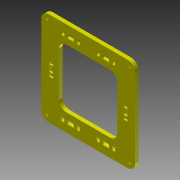
# Autodesk Inventor part: base
Saved by Autodesk Inventor 2012 SP1 (Build 160190100, 190)
## iProperties
Created: 2011-10-14
Part Number: base
Document SubType Name: Modeling
Designer: cramera
Density: 0.952 g/cm^3
Material: High Density Polyethylene
Mass: 589.682 g
Surface Area: 1422.26 cm^2
Volume: 619.414 cm^3
Autodesk Inventor part; units mm, degrees
ref_plane "YZ Plane" through (0, 0, 0) normal (1, 0, 0) x (0, 1, 0)
ref_plane "XZ Plane" through (0, 0, 0) normal (0, 1, 0) x (-1, 0, 0)
ref_plane "XY Plane" through (0, 0, 0) normal (0, 0, 1) x (1, 0, 0)
derived "skeleton.ipt"
sketch "POCKET_1-4" plane through (0, 0, 0) normal (0, 0, 1) x (1, 0, 0)
  line L0 (756.4523, 867.4563) -> (756.4523, 854.7563)
  arc A0 (791.01, 767.5708) -> (789.4225, 769.1583) centre (789.4225, 767.5708) ccw
  arc A1 (683.1733, 854.7563) -> (684.7608, 853.1688) centre (684.7608, 854.7563) ccw
  line L1 (683.1733, 854.7563) -> (683.1733, 867.4563)
  arc A2 (684.7608, 869.0438) -> (683.1733, 867.4563) centre (684.7608, 867.4563) ccw
  line L2 (684.7608, 869.0438) -> (754.8648, 869.0438)
  line L3 (756.4523, 613.4563) -> (756.4523, 626.1563)
  arc A3 (684.7608, 627.7438) -> (683.1733, 626.1563) centre (684.7608, 626.1563) ccw
  line L4 (683.1733, 626.1563) -> (683.1733, 613.4563)
  arc A4 (683.1733, 613.4563) -> (684.7608, 611.8688) centre (684.7608, 613.4563) ccw
  line L5 (684.7608, 611.8688) -> (754.8648, 611.8688)
  arc A5 (754.8648, 611.8688) -> (756.4523, 613.4563) centre (754.8648, 613.4563) ccw
  arc A6 (756.4523, 867.4563) -> (754.8648, 869.0438) centre (754.8648, 867.4563) ccw
  arc A7 (756.4523, 626.1563) -> (754.8648, 627.7438) centre (754.8648, 626.1563) ccw
  line L6 (754.8648, 627.7438) -> (684.7608, 627.7438)
  arc A8 (789.4225, 711.7543) -> (791.01, 713.3418) centre (789.4225, 713.3418) ccw
  line L7 (789.4225, 711.7543) -> (776.7225, 711.7543)
  arc A9 (775.135, 713.3418) -> (776.7225, 711.7543) centre (776.7225, 713.3418) ccw
  line L8 (775.135, 713.3418) -> (775.135, 767.5708)
  arc A10 (776.7225, 769.1583) -> (775.135, 767.5708) centre (776.7225, 767.5708) ccw
  line L9 (776.7225, 769.1583) -> (789.4225, 769.1583)
  line L10 (791.01, 767.5708) -> (791.01, 713.3418)
  arc A11 (568.3926, 613.4563) -> (569.9801, 611.8688) centre (569.9801, 613.4563) ccw
  line L11 (568.3926, 613.4563) -> (568.3926, 626.1563)
  arc A12 (569.9801, 627.7438) -> (568.3926, 626.1563) centre (569.9801, 626.1563) ccw
  line L12 (569.9801, 627.7438) -> (640.0841, 627.7438)
  arc A13 (641.6716, 626.1563) -> (640.0841, 627.7438) centre (640.0841, 626.1563) ccw
  line L13 (641.6716, 626.1563) -> (641.6716, 613.4563)
  arc A14 (640.0841, 611.8688) -> (641.6716, 613.4563) centre (640.0841, 613.4563) ccw
  line L14 (640.0841, 611.8688) -> (569.9801, 611.8688)
  arc A15 (641.6716, 867.4563) -> (640.0841, 869.0438) centre (640.0841, 867.4563) ccw
  line L15 (640.0841, 869.0438) -> (569.9801, 869.0438)
  arc A16 (569.9801, 869.0438) -> (568.3926, 867.4563) centre (569.9801, 867.4563) ccw
  line L16 (568.3926, 867.4563) -> (568.3926, 854.7563)
  arc A17 (568.3926, 854.7563) -> (569.9801, 853.1688) centre (569.9801, 854.7563) ccw
  line L17 (569.9801, 853.1688) -> (640.0841, 853.1688)
  arc A18 (640.0841, 853.1688) -> (641.6716, 854.7563) centre (640.0841, 854.7563) ccw
  line L18 (641.6716, 854.7563) -> (641.6716, 867.4563)
  arc A19 (533.835, 713.3418) -> (535.4225, 711.7543) centre (535.4225, 713.3418) ccw
  line L19 (535.4225, 711.7543) -> (548.1225, 711.7543)
  arc A20 (548.1225, 711.7543) -> (549.71, 713.3418) centre (548.1225, 713.3418) ccw
  line L20 (549.71, 713.3418) -> (549.71, 767.5708)
  arc A21 (549.71, 767.5708) -> (548.1225, 769.1583) centre (548.1225, 767.5708) ccw
  line L21 (548.1225, 769.1583) -> (535.4225, 769.1583)
  arc A22 (535.4225, 769.1583) -> (533.835, 767.5708) centre (535.4225, 767.5708) ccw
  line L22 (533.835, 767.5708) -> (533.835, 713.3418)
  arc A23 (754.8648, 853.1688) -> (756.4523, 854.7563) centre (754.8648, 854.7563) ccw
  line L23 (754.8648, 853.1688) -> (684.7608, 853.1688)
  constraints: 48 end point, 48 point on circle, 24 centre point
sketch "STOCK_12MM" plane through (0, 0, 0) normal (0, 0, 1) x (1, 0, 0)
  line L0 (457.2, 0) -> (914.4, 0)
  line L1 (914.4, 0) -> (914.4, 914.4)
  line L2 (914.4, 914.4) -> (457.2, 914.4)
  line L3 (457.2, 914.4) -> (457.2, 0)
  line L4 (457.2, 0) -> (457.2, 914.4)
  constraints: 10 end point
sketch "THROUGH-CUT" plane through (0, 0, 0) normal (0, 0, 1) x (1, 0, 0)
  arc A0 (777.1035, 720.3494) -> (779.3485, 718.1043) centre (778.226, 719.2268) ccw
  line L0 (779.3485, 718.1043) -> (787.1774, 718.1043)
  arc A1 (787.1774, 718.1043) -> (789.4225, 720.3494) centre (788.2999, 719.2268) ccw
  line L1 (789.4225, 720.3494) -> (789.4225, 726.0192)
  arc A2 (594.5546, 613.4563) -> (596.7997, 613.4563) centre (595.6772, 614.5788) ccw
  line L2 (596.7997, 613.4563) -> (613.2646, 613.4563)
  arc A3 (613.2646, 613.4563) -> (615.5096, 613.4563) centre (614.3871, 614.5788) ccw
  arc A4 (615.5096, 613.4563) -> (615.5096, 615.7014) centre (614.3871, 614.5788) ccw
  line L3 (615.5096, 615.7014) -> (615.5096, 623.5302)
  arc A5 (615.5096, 623.5302) -> (615.5096, 625.7753) centre (614.3871, 624.6528) ccw
  arc A6 (615.5096, 625.7753) -> (613.2646, 625.7753) centre (614.3871, 624.6528) ccw
  line L4 (613.2646, 625.7753) -> (596.7997, 625.7753)
  arc A7 (596.7997, 625.7753) -> (594.5546, 623.5302) centre (595.6772, 624.6528) ccw
  line L5 (594.5546, 623.5302) -> (594.5546, 615.7014)
  arc A8 (594.5546, 615.7014) -> (594.5546, 613.4563) centre (595.6772, 614.5788) ccw
  arc A9 (728.0452, 613.4563) -> (730.2903, 613.4563) centre (729.1678, 614.5788) ccw
  line L6 (728.0452, 613.4563) -> (711.5804, 613.4563)
  arc A10 (709.3353, 613.4563) -> (711.5804, 613.4563) centre (710.4578, 614.5788) ccw
  arc A11 (709.3353, 615.7014) -> (709.3353, 613.4563) centre (710.4578, 614.5788) ccw
  line L7 (709.3353, 615.7014) -> (709.3353, 623.5302)
  arc A12 (709.3353, 625.7753) -> (709.3353, 623.5302) centre (710.4578, 624.6528) ccw
  arc A13 (711.5804, 625.7753) -> (709.3353, 625.7753) centre (710.4578, 624.6528) ccw
  line L8 (711.5804, 625.7753) -> (728.0452, 625.7753)
  arc A14 (730.2903, 623.5302) -> (728.0452, 625.7753) centre (729.1678, 624.6528) ccw
  line L9 (730.2903, 623.5302) -> (730.2903, 615.7014)
  arc A15 (730.2903, 613.4563) -> (730.2903, 615.7014) centre (729.1678, 614.5788) ccw
  arc A16 (625.1616, 855.1373) -> (627.4067, 855.1373) centre (626.2842, 856.2598) ccw
  arc A17 (625.1616, 857.3824) -> (625.1616, 855.1373) centre (626.2842, 856.2598) ccw
  line L10 (625.1616, 857.3824) -> (625.1616, 865.2112)
  arc A18 (625.1616, 867.4563) -> (625.1616, 865.2112) centre (626.2842, 866.3338) ccw
  arc A19 (627.4067, 867.4563) -> (625.1616, 867.4563) centre (626.2842, 866.3338) ccw
  line L11 (627.4067, 867.4563) -> (633.0766, 867.4563)
  arc A20 (635.3216, 867.4563) -> (633.0766, 867.4563) centre (634.1991, 866.3338) ccw
  arc A21 (635.3216, 865.2112) -> (635.3216, 867.4563) centre (634.1991, 866.3338) ccw
  line L12 (635.3216, 865.2112) -> (635.3216, 857.3824)
  arc A22 (635.3216, 855.1373) -> (635.3216, 857.3824) centre (634.1991, 856.2598) ccw
  arc A23 (633.0766, 855.1373) -> (635.3216, 855.1373) centre (634.1991, 856.2598) ccw
  line L13 (633.0766, 855.1373) -> (627.4067, 855.1373)
  arc A24 (627.4067, 625.7753) -> (625.1616, 625.7753) centre (626.2842, 624.6528) ccw
  arc A25 (625.1616, 625.7753) -> (625.1616, 623.5302) centre (626.2842, 624.6528) ccw
  line L14 (625.1616, 623.5302) -> (625.1616, 615.7014)
  arc A26 (625.1616, 615.7014) -> (625.1616, 613.4563) centre (626.2842, 614.5788) ccw
  arc A27 (625.1616, 613.4563) -> (627.4067, 613.4563) centre (626.2842, 614.5788) ccw
  line L15 (627.4067, 613.4563) -> (633.0766, 613.4563)
  arc A28 (633.0766, 613.4563) -> (635.3216, 613.4563) centre (634.1991, 614.5788) ccw
  arc A29 (635.3216, 613.4563) -> (635.3216, 615.7014) centre (634.1991, 614.5788) ccw
  line L16 (635.3216, 615.7014) -> (635.3216, 623.5302)
  arc A30 (635.3216, 623.5302) -> (635.3216, 625.7753) centre (634.1991, 624.6528) ccw
  arc A31 (635.3216, 625.7753) -> (633.0766, 625.7753) centre (634.1991, 624.6528) ccw
  line L17 (633.0766, 625.7753) -> (627.4067, 625.7753)
  arc A32 (697.4382, 855.1373) -> (699.6833, 855.1373) centre (698.5608, 856.2598) ccw
  arc A33 (699.6833, 855.1373) -> (699.6833, 857.3824) centre (698.5608, 856.2598) ccw
  line L18 (699.6833, 857.3824) -> (699.6833, 865.2112)
  arc A34 (699.6833, 865.2112) -> (699.6833, 867.4563) centre (698.5608, 866.3338) ccw
  arc A35 (699.6833, 867.4563) -> (697.4382, 867.4563) centre (698.5608, 866.3338) ccw
  line L19 (697.4382, 867.4563) -> (691.7684, 867.4563)
  arc A36 (691.7684, 867.4563) -> (689.5233, 867.4563) centre (690.6458, 866.3338) ccw
  arc A37 (689.5233, 867.4563) -> (689.5233, 865.2112) centre (690.6458, 866.3338) ccw
  line L20 (689.5233, 865.2112) -> (689.5233, 857.3824)
  arc A38 (689.5233, 857.3824) -> (689.5233, 855.1373) centre (690.6458, 856.2598) ccw
  arc A39 (689.5233, 855.1373) -> (691.7684, 855.1373) centre (690.6458, 856.2598) ccw
  line L21 (691.7684, 855.1373) -> (697.4382, 855.1373)
  arc A40 (574.7426, 857.3824) -> (574.7426, 855.1373) centre (575.8652, 856.2598) ccw
  line L22 (574.7426, 857.3824) -> (574.7426, 865.2112)
  arc A41 (574.7426, 867.4563) -> (574.7426, 865.2112) centre (575.8652, 866.3338) ccw
  arc A42 (576.9877, 867.4563) -> (574.7426, 867.4563) centre (575.8652, 866.3338) ccw
  line L23 (576.9877, 867.4563) -> (582.6576, 867.4563)
  arc A43 (584.9026, 867.4563) -> (582.6576, 867.4563) centre (583.7801, 866.3338) ccw
  arc A44 (584.9026, 865.2112) -> (584.9026, 867.4563) centre (583.7801, 866.3338) ccw
  line L24 (584.9026, 865.2112) -> (584.9026, 857.3824)
  arc A45 (584.9026, 855.1373) -> (584.9026, 857.3824) centre (583.7801, 856.2598) ccw
  arc A46 (582.6576, 855.1373) -> (584.9026, 855.1373) centre (583.7801, 856.2598) ccw
  line L25 (582.6576, 855.1373) -> (576.9877, 855.1373)
  arc A47 (574.7426, 855.1373) -> (576.9877, 855.1373) centre (575.8652, 856.2598) ccw
  arc A48 (750.1023, 855.1373) -> (750.1023, 857.3824) centre (748.9798, 856.2598) ccw
  line L26 (750.1023, 857.3824) -> (750.1023, 865.2112)
  arc A49 (750.1023, 865.2112) -> (750.1023, 867.4563) centre (748.9798, 866.3338) ccw
  arc A50 (750.1023, 867.4563) -> (747.8572, 867.4563) centre (748.9798, 866.3338) ccw
  line L27 (747.8572, 867.4563) -> (742.1874, 867.4563)
  arc A51 (742.1874, 867.4563) -> (739.9423, 867.4563) centre (741.0648, 866.3338) ccw
  arc A52 (739.9423, 867.4563) -> (739.9423, 865.2112) centre (741.0648, 866.3338) ccw
  arc A53 (545.4964, 718.1043) -> (547.7415, 720.3494) centre (546.6189, 719.2268) ccw
  arc A54 (739.9423, 857.3824) -> (739.9423, 855.1373) centre (741.0648, 856.2598) ccw
  arc A55 (739.9423, 855.1373) -> (742.1874, 855.1373) centre (741.0648, 856.2598) ccw
  line L28 (742.1874, 855.1373) -> (747.8572, 855.1373)
  arc A56 (747.8572, 855.1373) -> (750.1023, 855.1373) centre (748.9798, 856.2598) ccw
  arc A57 (750.1023, 623.5302) -> (750.1023, 625.7753) centre (748.9798, 624.6528) ccw
  line L29 (750.1023, 623.5302) -> (750.1023, 615.7014)
  arc A58 (750.1023, 613.4563) -> (750.1023, 615.7014) centre (748.9798, 614.5788) ccw
  arc A59 (747.8572, 613.4563) -> (750.1023, 613.4563) centre (748.9798, 614.5788) ccw
  line L30 (747.8572, 613.4563) -> (742.1874, 613.4563)
  arc A60 (739.9423, 613.4563) -> (742.1874, 613.4563) centre (741.0648, 614.5788) ccw
  arc A61 (739.9423, 615.7014) -> (739.9423, 613.4563) centre (741.0648, 614.5788) ccw
  line L31 (739.9423, 615.7014) -> (739.9423, 623.5302)
  arc A62 (739.9423, 625.7753) -> (739.9423, 623.5302) centre (741.0648, 624.6528) ccw
  arc A63 (742.1874, 625.7753) -> (739.9423, 625.7753) centre (741.0648, 624.6528) ccw
  line L32 (742.1874, 625.7753) -> (747.8572, 625.7753)
  arc A64 (750.1023, 625.7753) -> (747.8572, 625.7753) centre (748.9798, 624.6528) ccw
  circle A65 centre (527.8454, 605.8792) radius 3.175
  arc A66 (574.7426, 625.7753) -> (574.7426, 623.5302) centre (575.8652, 624.6528) ccw
  line L33 (574.7426, 623.5302) -> (574.7426, 615.7014)
  arc A67 (574.7426, 615.7014) -> (574.7426, 613.4563) centre (575.8652, 614.5788) ccw
  arc A68 (574.7426, 613.4563) -> (576.9877, 613.4563) centre (575.8652, 614.5788) ccw
  line L34 (576.9877, 613.4563) -> (582.6576, 613.4563)
  arc A69 (582.6576, 613.4563) -> (584.9026, 613.4563) centre (583.7801, 614.5788) ccw
  arc A70 (584.9026, 613.4563) -> (584.9026, 615.7014) centre (583.7801, 614.5788) ccw
  line L35 (584.9026, 615.7014) -> (584.9026, 623.5302)
  arc A71 (584.9026, 623.5302) -> (584.9026, 625.7753) centre (583.7801, 624.6528) ccw
  arc A72 (584.9026, 625.7753) -> (582.6576, 625.7753) centre (583.7801, 624.6528) ccw
  line L36 (582.6576, 625.7753) -> (576.9877, 625.7753)
  arc A73 (576.9877, 625.7753) -> (574.7426, 625.7753) centre (575.8652, 624.6528) ccw
  circle A74 centre (796.9996, 875.0334) radius 3.175
  arc A75 (596.7997, 867.4563) -> (594.5546, 867.4563) centre (595.6772, 866.3338) ccw
  line L37 (596.7997, 867.4563) -> (613.2646, 867.4563)
  arc A76 (615.5096, 867.4563) -> (613.2646, 867.4563) centre (614.3871, 866.3338) ccw
  arc A77 (615.5096, 865.2112) -> (615.5096, 867.4563) centre (614.3871, 866.3338) ccw
  line L38 (615.5096, 865.2112) -> (615.5096, 857.3824)
  arc A78 (615.5096, 855.1373) -> (615.5096, 857.3824) centre (614.3871, 856.2598) ccw
  arc A79 (613.2646, 855.1373) -> (615.5096, 855.1373) centre (614.3871, 856.2598) ccw
  line L39 (613.2646, 855.1373) -> (596.7997, 855.1373)
  arc A80 (594.5546, 857.3824) -> (596.7997, 855.1373) centre (595.6772, 856.2598) ccw
  line L40 (594.5546, 857.3824) -> (594.5546, 865.2112)
  arc A81 (594.5546, 867.4563) -> (594.5546, 865.2112) centre (595.6772, 866.3338) ccw
  circle A82 centre (527.8454, 875.0334) radius 3.175
  circle A83 centre (796.9996, 605.8792) radius 3.175
  line L41 (787.1774, 762.8083) -> (779.3485, 762.8083)
  arc A84 (779.3485, 762.8083) -> (777.1035, 760.5632) centre (778.226, 761.6858) ccw
  line L42 (777.1035, 760.5632) -> (777.1035, 754.8934)
  arc A85 (777.1035, 754.8934) -> (777.1035, 752.6483) centre (778.226, 753.7708) ccw
  arc A86 (777.1035, 752.6483) -> (779.3485, 752.6483) centre (778.226, 753.7708) ccw
  line L43 (779.3485, 752.6483) -> (787.1774, 752.6483)
  arc A87 (787.1774, 752.6483) -> (789.4225, 752.6483) centre (788.2999, 753.7708) ccw
  arc A88 (789.4225, 752.6483) -> (789.4225, 754.8934) centre (788.2999, 753.7708) ccw
  line L44 (789.4225, 754.8934) -> (789.4225, 760.5632)
  arc A89 (789.4225, 760.5632) -> (787.1774, 762.8083) centre (788.2999, 761.6858) ccw
  line L45 (732.2725, 835.7063) -> (592.5725, 835.7063)
  arc A90 (592.5725, 835.7063) -> (567.1725, 810.3063) centre (592.5725, 810.3063) ccw
  line L46 (567.1725, 810.3063) -> (567.1725, 670.6063)
  arc A91 (567.1725, 670.6063) -> (592.5725, 645.2063) centre (592.5725, 670.6063) ccw
  line L47 (592.5725, 645.2063) -> (732.2725, 645.2063)
  arc A92 (732.2725, 645.2063) -> (757.6725, 670.6063) centre (732.2725, 670.6063) ccw
  line L48 (757.6725, 670.6063) -> (757.6725, 810.3063)
  arc A93 (757.6725, 810.3063) -> (732.2725, 835.7063) centre (732.2725, 810.3063) ccw
  line L49 (547.7415, 747.1012) -> (547.7415, 733.8114)
  arc A94 (547.7415, 731.5663) -> (547.7415, 733.8114) centre (546.6189, 732.6888) ccw
  arc A95 (545.4964, 731.5663) -> (547.7415, 731.5663) centre (546.6189, 732.6888) ccw
  line L50 (545.4964, 731.5663) -> (537.6675, 731.5663)
  arc A96 (535.4225, 731.5663) -> (537.6675, 731.5663) centre (536.545, 732.6888) ccw
  arc A97 (535.4225, 733.8114) -> (535.4225, 731.5663) centre (536.545, 732.6888) ccw
  arc A98 (730.2903, 867.4563) -> (728.0452, 867.4563) centre (729.1678, 866.3338) ccw
  arc A99 (537.6675, 749.3463) -> (535.4225, 747.1012) centre (536.545, 748.2238) ccw
  line L51 (537.6675, 749.3463) -> (545.4964, 749.3463)
  arc A100 (547.7415, 747.1012) -> (545.4964, 749.3463) centre (546.6189, 748.2238) ccw
  line L52 (728.0452, 867.4563) -> (711.5804, 867.4563)
  arc A101 (711.5804, 867.4563) -> (709.3353, 867.4563) centre (710.4578, 866.3338) ccw
  arc A102 (709.3353, 867.4563) -> (709.3353, 865.2112) centre (710.4578, 866.3338) ccw
  line L53 (709.3353, 865.2112) -> (709.3353, 857.3824)
  line L54 (777.1035, 747.1012) -> (777.1035, 733.8114)
  arc A103 (777.1035, 733.8114) -> (777.1035, 731.5663) centre (778.226, 732.6888) ccw
  arc A104 (777.1035, 731.5663) -> (779.3485, 731.5663) centre (778.226, 732.6888) ccw
  line L55 (779.3485, 731.5663) -> (787.1774, 731.5663)
  arc A105 (787.1774, 731.5663) -> (789.4225, 731.5663) centre (788.2999, 732.6888) ccw
  arc A106 (789.4225, 731.5663) -> (789.4225, 733.8114) centre (788.2999, 732.6888) ccw
  line L56 (789.4225, 733.8114) -> (789.4225, 747.1012)
  arc A107 (789.4225, 747.1012) -> (787.1774, 749.3463) centre (788.2999, 748.2238) ccw
  line L57 (787.1774, 749.3463) -> (779.3485, 749.3463)
  arc A108 (779.3485, 749.3463) -> (777.1035, 747.1012) centre (778.226, 748.2238) ccw
  arc A109 (709.3353, 857.3824) -> (709.3353, 855.1373) centre (710.4578, 856.2598) ccw
  arc A110 (709.3353, 855.1373) -> (711.5804, 855.1373) centre (710.4578, 856.2598) ccw
  line L58 (711.5804, 855.1373) -> (728.0452, 855.1373)
  arc A111 (728.0452, 855.1373) -> (730.2903, 857.3824) centre (729.1678, 856.2598) ccw
  line L59 (730.2903, 857.3824) -> (730.2903, 865.2112)
  arc A112 (730.2903, 865.2112) -> (730.2903, 867.4563) centre (729.1678, 866.3338) ccw
  line L60 (537.6675, 762.8083) -> (545.4964, 762.8083)
  arc A113 (547.7415, 760.5632) -> (545.4964, 762.8083) centre (546.6189, 761.6858) ccw
  line L61 (547.7415, 760.5632) -> (547.7415, 754.8934)
  arc A114 (547.7415, 752.6483) -> (547.7415, 754.8934) centre (546.6189, 753.7708) ccw
  arc A115 (545.4964, 752.6483) -> (547.7415, 752.6483) centre (546.6189, 753.7708) ccw
  line L62 (545.4964, 752.6483) -> (537.6675, 752.6483)
  arc A116 (535.4225, 752.6483) -> (537.6675, 752.6483) centre (536.545, 753.7708) ccw
  arc A117 (535.4225, 754.8934) -> (535.4225, 752.6483) centre (536.545, 753.7708) ccw
  line L63 (535.4225, 754.8934) -> (535.4225, 760.5632)
  line L64 (739.9423, 865.2112) -> (739.9423, 857.3824)
  arc A118 (537.6675, 762.8083) -> (535.4225, 760.5632) centre (536.545, 761.6858) ccw
  line L65 (535.4225, 588.0563) -> (789.4225, 588.0563)
  arc A119 (789.4225, 588.0563) -> (814.8225, 613.4563) centre (789.4225, 613.4563) ccw
  line L66 (814.8225, 613.4563) -> (814.8225, 867.4563)
  arc A120 (814.8225, 867.4563) -> (789.4225, 892.8563) centre (789.4225, 867.4563) ccw
  line L67 (789.4225, 892.8563) -> (535.4225, 892.8563)
  arc A121 (535.4225, 892.8563) -> (510.0225, 867.4563) centre (535.4225, 867.4563) ccw
  line L68 (510.0225, 867.4563) -> (510.0225, 613.4563)
  arc A122 (510.0225, 613.4563) -> (535.4225, 588.0563) centre (535.4225, 613.4563) ccw
  arc A123 (537.6675, 728.2643) -> (535.4225, 726.0192) centre (536.545, 727.1418) ccw
  line L69 (537.6675, 728.2643) -> (545.4964, 728.2643)
  arc A124 (547.7415, 726.0192) -> (545.4964, 728.2643) centre (546.6189, 727.1418) ccw
  line L70 (547.7415, 726.0192) -> (547.7415, 720.3494)
  line L71 (545.4964, 718.1043) -> (537.6675, 718.1043)
  arc A125 (535.4225, 720.3494) -> (537.6675, 718.1043) centre (536.545, 719.2268) ccw
  line L72 (535.4225, 720.3494) -> (535.4225, 726.0192)
  arc A126 (699.6833, 625.7753) -> (697.4382, 625.7753) centre (698.5608, 624.6528) ccw
  arc A127 (699.6833, 623.5302) -> (699.6833, 625.7753) centre (698.5608, 624.6528) ccw
  line L73 (699.6833, 623.5302) -> (699.6833, 615.7014)
  arc A128 (699.6833, 613.4563) -> (699.6833, 615.7014) centre (698.5608, 614.5788) ccw
  arc A129 (697.4382, 613.4563) -> (699.6833, 613.4563) centre (698.5608, 614.5788) ccw
  line L74 (697.4382, 613.4563) -> (691.7684, 613.4563)
  arc A130 (689.5233, 613.4563) -> (691.7684, 613.4563) centre (690.6458, 614.5788) ccw
  arc A131 (689.5233, 615.7014) -> (689.5233, 613.4563) centre (690.6458, 614.5788) ccw
  line L75 (689.5233, 615.7014) -> (689.5233, 623.5302)
  arc A132 (689.5233, 625.7753) -> (689.5233, 623.5302) centre (690.6458, 624.6528) ccw
  arc A133 (691.7684, 625.7753) -> (689.5233, 625.7753) centre (690.6458, 624.6528) ccw
  line L76 (691.7684, 625.7753) -> (697.4382, 625.7753)
  arc A134 (789.4225, 726.0192) -> (787.1774, 728.2643) centre (788.2999, 727.1418) ccw
  line L77 (787.1774, 728.2643) -> (779.3485, 728.2643)
  arc A135 (779.3485, 728.2643) -> (777.1035, 726.0192) centre (778.226, 727.1418) ccw
  line L78 (777.1035, 726.0192) -> (777.1035, 720.3494)
  line L79 (535.4225, 733.8114) -> (535.4225, 747.1012)
  constraints: 264 point on circle, 160 end point, 136 centre point
extrude "Extrusion1" add sketch "THROUGH-CUT" along normal blind 12
extrude "Extrusion2" cut sketch "POCKET_1-4" along normal blind 6.35
equation "\"d1\" = StockThickness"
equation "\"StockThickness\" = 12"
body "Solid1"
